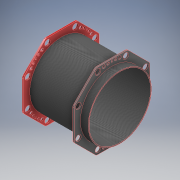
# Autodesk Inventor part: Primary
Saved by Autodesk Inventor 2022 (Build 260153000, 153)
## iProperties
Created: 2021-04-24
Part Number: Primary
Material: Generic
Document SubType Name: Modeling
Designer: Mick Veldhuis
Density: 1 g/cm^3
Appearance: Red
Author: Mick Veldhuis
Autodesk Inventor part; units mm, degrees
ref_plane "YZ Plane" through (0, 0, 0) normal (1, 0, 0) x (0, 1, 0)
sketch "Sketch1" plane through (0, 0, 0) normal (1, 0, 0) x (0, 1, 0)
  circle A0 centre (0, 0) radius 200
  constraints: 1 centre point, 1 coincident
extrude "Extrusion1" add sketch "Sketch1" along normal blind 370
sketch "Sketch2" plane through (0, 0, 0) normal (-1, 0, 0) x (0, 0, 1)
  point P0 (0, 0)
sketch "Sketch3" plane through (370, 0, 0) normal (1, 0, 0) x (0, 0, -1)
  circle A0 centre (0, 0) radius 195
  dimension "d2" = 390
  constraints: 1 centre point, 1 coincident
  measures "d2" diameter of A0
extrude "Extrusion2" cut sketch "Sketch3" against normal blind 370
ref_plane "Work Plane1" through (0, 0, 0) normal (-1, 0, 0) x (0, 0, 1)
sketch "Sketch4" plane through (0, 0, 0) normal (-1, 0, 0) x (0, 0, 1)
  point P0 (0, 0)
sketch "Sketch5" plane through (0, 0, 0) normal (-1, 0, 0) x (0, 0, 1)
  line L0 (240, -99.4113) -> (99.4113, -240)
  line L1 (99.4113, -240) -> (-99.4113, -240)
  line L2 (-99.4113, -240) -> (-240, -99.4113)
  line L3 (-240, -99.4113) -> (-240, 99.4113)
  line L4 (-240, 99.4113) -> (-99.4113, 240)
  line L5 (-99.4113, 240) -> (99.4113, 240)
  line L6 (99.4113, 240) -> (240, 99.4113)
  line L7 (240, 99.4113) -> (240, -99.4113)
  point P0 (0, 0)
  point P1 (0, 0)
  constraints: 16 end point, 1 coincident, 17 other
extrude "BackPlate" add sketch "Sketch5" along normal blind 8
fillet "Fillet1" radius 20 8 edges at (-4, -240, 99.4113) (-4, -240, -99.4113) (-4, -99.4113, -240) (-4, 99.4113, -240) (-4, 240, -99.4113) (-4, 240, 99.4113) (-4, 99.4113, 240) (-4, -99.4113, 240)
ref_plane "Work Plane3" through (320, 0, 0) normal (-1, 0, 0) x (0, 0, 1)
sketch "Sketch6" plane through (320, 0, 0) normal (-1, 0, 0) x (0, 0, 1)
  line L0 (91.127, 240) -> (-91.127, 240) projected
  line L1 (99.4113, 240) -> (240, 99.4113)
  line L2 (240, 99.4113) -> (240, -99.4113)
  line L3 (240, -99.4113) -> (99.4113, -240)
  line L4 (99.4113, -240) -> (-99.4113, -240)
  line L5 (-99.4113, -240) -> (-240, -99.4113)
  line L6 (-240, -99.4113) -> (-240, 99.4113)
  line L7 (-240, 99.4113) -> (-99.4113, 240)
  line L8 (-99.4113, 240) -> (99.4113, 240)
  point P0 (0, 0)
  point P1 (0, 0)
  point P2 (0, 240)
  constraints: 16 end point, 2 midpoint, 1 coincident, 17 other
extrude "FrontPlate" add sketch "Sketch6" along normal blind 8
sketch "Sketch7" plane through (320, 0, 0) normal (1, 0, 0) x (0, 0, -1)
  circle A0 centre (0, 0) radius 195
  constraints: 1 centre point, 1 coincident
extrude "Extrusion5" cut sketch "Sketch7" against normal blind 8
fillet "Fillet2" radius 20 8 edges at (316, -99.4113, 240) (316, 99.4113, 240) (316, 240, 99.4113) (316, 240, -99.4113) (316, 99.4113, -240) (316, -99.4113, -240) (316, -240, -99.4113) (316, -240, 99.4113)
sketch "BackplateHoles" plane through (0, 0, 0) normal (1, 0, 0) x (0, 0, -1)
  circle A0 centre (-88, 212) radius 18
  circle A1 centre (-88, -212) radius 18
  circle A2 centre (-212, 88) radius 18
  circle A3 centre (-212, -88) radius 18
  circle A4 centre (-190, 122) radius 10
  circle A5 centre (-122, 190) radius 10
  circle A6 centre (-144, 176) radius 8
  circle A7 centre (-176, 144) radius 8
  circle A8 centre (-162, 162) radius 6
  line L0 (-240, 0) -> (240, 0) construction
  circle A9 centre (-190, -122) radius 10
  circle A10 centre (-176, -144) radius 8
  circle A11 centre (-162, -162) radius 6
  circle A12 centre (-144, -176) radius 8
  circle A13 centre (-122, -190) radius 10
  circle A14 centre (88, 212) radius 18
  circle A15 centre (212, 88) radius 18
  circle A16 centre (190, 122) radius 10
  circle A17 centre (122, 190) radius 10
  circle A18 centre (144, 176) radius 8
  circle A19 centre (176, 144) radius 8
  circle A20 centre (162, 162) radius 6
  circle A21 centre (88, -212) radius 18
  circle A22 centre (212, -88) radius 18
  circle A23 centre (190, -122) radius 10
  circle A24 centre (162, -162) radius 6
  circle A25 centre (144, -176) radius 8
  circle A26 centre (122, -190) radius 10
  circle A27 centre (176, -144) radius 8
  point P0 (0, 0)
  point P1 (0, 0)
  constraints: 28 centre point, 6 coincident, 6 symmetric about line, 2 end point, 5 other
sketch "FrontplateHoles" plane through (320, 0, 0) normal (1, 0, 0) x (0, 0, -1)
  circle A0 centre (-88, 212) radius 18
  circle A1 centre (-88, -212) radius 18
  circle A2 centre (-212, 88) radius 18
  circle A3 centre (-212, -88) radius 18
  circle A4 centre (-190, 122) radius 10
  circle A5 centre (-122, 190) radius 10
  circle A6 centre (-144, 176) radius 8
  circle A7 centre (-176, 144) radius 8
  circle A8 centre (-162, 162) radius 6
  circle A9 centre (50, -222) radius 10
  circle A10 centre (24, -226) radius 8
  circle A11 centre (0, -228) radius 6
  circle A12 centre (-24, -226) radius 8
  circle A13 centre (-50, -222) radius 10
  circle A14 centre (-190, -122) radius 10
  circle A15 centre (-176, -144) radius 8
  circle A16 centre (-162, -162) radius 6
  circle A17 centre (-144, -176) radius 8
  circle A18 centre (-122, -190) radius 10
  circle A19 centre (88, 212) radius 18
  circle A20 centre (212, 88) radius 18
  circle A21 centre (190, 122) radius 10
  circle A22 centre (122, 190) radius 10
  circle A23 centre (144, 176) radius 8
  circle A24 centre (176, 144) radius 8
  circle A25 centre (162, 162) radius 6
  circle A26 centre (88, -212) radius 18
  circle A27 centre (212, -88) radius 18
  circle A28 centre (190, -122) radius 10
  circle A29 centre (162, -162) radius 6
  circle A30 centre (144, -176) radius 8
  circle A31 centre (122, -190) radius 10
  circle A32 centre (176, -144) radius 8
  circle A33 centre (222.0138, -50) radius 10
  circle A34 centre (226, -24) radius 8
  circle A35 centre (228.0138, 0) radius 6
  circle A36 centre (226, 24) radius 8
  circle A37 centre (222.0138, 50) radius 10
  circle A38 centre (-222, -50) radius 10
  circle A39 centre (-226, -24) radius 8
  circle A40 centre (-228, 0) radius 6
  circle A41 centre (-226, 24) radius 8
  circle A42 centre (-222, 50) radius 10
  circle A43 centre (50, 222) radius 10
  circle A44 centre (24, 226) radius 8
  circle A45 centre (0, 228) radius 6
  circle A46 centre (-24, 226) radius 8
  circle A47 centre (-50, 222) radius 10
  point P0 (0, 0)
  point P1 (0, 0)
  constraints: 48 centre point, 20 coincident
hole "Hole1" at (0, -212, -88) at (0, -88, -212) at (0, 88, -212) at (0, 212, -88) at (0, 212, 88) at (0, 88, 212) at (0, -88, 212) at (0, -212, 88) direction (-1, 0, 0) diameter 36 depth 8
hole "Hole2" at (0, -190, 122) at (0, -122, 190) at (0, 122, 190) at (0, 190, 122) at (0, 190, -122) at (0, 122, -190) at (0, -122, -190) at (0, -190, -122) direction (-1, 0, 0) diameter 20 depth 8
hole "Hole3" at (0, -144, 176) at (0, 176, 144) at (0, 144, 176) at (0, -176, 144) at (0, -176, -144) at (0, -144, -176) at (0, 144, -176) at (0, 176, -144) direction (-1, 0, 0) diameter 16 depth 8
hole "Hole4" at (0, -162, 162) at (0, 162, 162) at (0, 162, -162) at (0, -162, -162) direction (-1, 0, 0) diameter 12 depth 8
hole "Hole5" at (320, -88, 212) at (320, 88, 212) at (320, 212, 88) at (320, 212, -88) at (320, -212, -88) at (320, -212, 88) at (320, -88, -212) at (320, 88, -212) direction (-1, 0, 0) diameter 36 depth 8
hole "Hole6" at (320, 222, 50) at (320, 222, -50) at (320, -222, 50) at (320, -222, -50) direction (-1, 0, 0) diameter 20 depth 8
hole "Hole7" at (320, -226, 24) at (320, -226, -24) at (320, 226, -24) at (320, 226, 24) direction (-1, 0, 0) diameter 16 depth 8
hole "Hole8" at (320, 228, 0) at (320, -228, 0) direction (-1, 0, 0) diameter 12 depth 8
body "Solid1"
